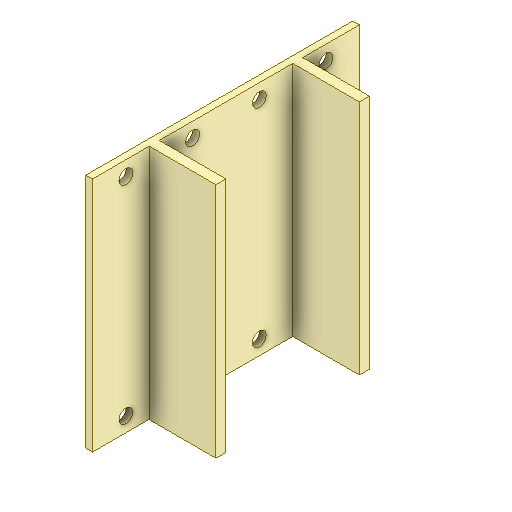
# Autodesk Inventor part: LegHolder
Saved by Autodesk Inventor 2022 (Build 260153000, 153)
## iProperties
Created: 2024-07-11
Part Number: LegHolder
Material: ABS Plastic
Document SubType Name: Modeling
Designer: LaptopJR
Density: 1.06 g/cm^3
Appearance: Nylon 6
Author: LaptopJR
Autodesk Inventor part; units mm, degrees
ref_plane "YZ Plane" through (0, 0, 0) normal (1, 0, 0) x (0, 1, 0)
ref_plane "XZ Plane" through (0, 0, 0) normal (0, 1, 0) x (-1, 0, 0)
ref_plane "Work Plane1" through (-4544.258, -3059.401, -4421.2024) normal (1, 0, 0) x (0, 1, 0)
sketch "Sketch1" plane through (-4544.258, -3059.401, -4421.2024) normal (1, 0, 0) x (0, 1, 0)
  line L0 (0.76, -160) -> (142.55, -160) projected
  line L1 (142.55, -160) -> (142.55, 0) projected
  line L2 (0.76, 0) -> (142.55, 0) projected
  line L3 (0.76, 0) -> (0.76, -160) projected
  arc A0 (9.505, -144.1656) -> (9.505, -135.8344) centre (9.505, -140) ccw projected
  arc A1 (9.505, -135.8344) -> (9.505, -144.1656) centre (9.505, -140) ccw projected
  arc A2 (133.805, -144.1656) -> (133.805, -135.8344) centre (133.805, -140) ccw projected
  arc A3 (133.805, -135.8344) -> (133.805, -144.1656) centre (133.805, -140) ccw projected
  arc A4 (133.805, -24.1656) -> (133.805, -15.8344) centre (133.805, -20) ccw projected
  arc A5 (133.805, -15.8344) -> (133.805, -24.1656) centre (133.805, -20) ccw projected
  arc A6 (9.505, -24.1656) -> (9.505, -15.8344) centre (9.505, -20) ccw projected
  arc A7 (9.505, -15.8344) -> (9.505, -24.1656) centre (9.505, -20) ccw projected
  arc A8 (51.655, -144.9403) -> (51.655, -135.0597) centre (51.655, -140) ccw construction
  arc A9 (51.655, -135.0597) -> (51.655, -144.9403) centre (51.655, -140) ccw construction
  arc A10 (51.655, -24.9403) -> (51.655, -15.0597) centre (51.655, -20) ccw construction
  arc A11 (51.655, -15.0597) -> (51.655, -24.9403) centre (51.655, -20) ccw construction
  arc A12 (91.655, -24.9403) -> (91.655, -15.0597) centre (91.655, -20) ccw construction
  arc A13 (91.655, -15.0597) -> (91.655, -24.9403) centre (91.655, -20) ccw construction
  arc A14 (9.505, -64.1656) -> (9.505, -55.8344) centre (9.505, -60) ccw projected
  arc A15 (9.505, -55.8344) -> (9.505, -64.1656) centre (9.505, -60) ccw projected
  arc A16 (9.505, -104.1656) -> (9.505, -95.8344) centre (9.505, -100) ccw projected
  arc A17 (9.505, -95.8344) -> (9.505, -104.1656) centre (9.505, -100) ccw projected
  arc A18 (133.805, -104.1656) -> (133.805, -95.8344) centre (133.805, -100) ccw projected
  arc A19 (133.805, -95.8344) -> (133.805, -104.1656) centre (133.805, -100) ccw projected
  arc A20 (133.805, -64.1656) -> (133.805, -55.8344) centre (133.805, -60) ccw projected
  arc A21 (133.805, -55.8344) -> (133.805, -64.1656) centre (133.805, -60) ccw projected
  arc A22 (51.655, -64.9403) -> (51.655, -55.0597) centre (51.655, -60) ccw construction
  arc A23 (51.655, -55.0597) -> (51.655, -64.9403) centre (51.655, -60) ccw construction
  arc A24 (51.655, -104.9403) -> (51.655, -95.0597) centre (51.655, -100) ccw construction
  arc A25 (51.655, -95.0597) -> (51.655, -104.9403) centre (51.655, -100) ccw construction
  arc A26 (91.655, -104.9403) -> (91.655, -95.0597) centre (91.655, -100) ccw construction
  arc A27 (91.655, -95.0597) -> (91.655, -104.9403) centre (91.655, -100) ccw construction
  arc A28 (91.655, -64.9403) -> (91.655, -55.0597) centre (91.655, -60) ccw construction
  arc A29 (91.655, -55.0597) -> (91.655, -64.9403) centre (91.655, -60) ccw construction
  arc A30 (91.655, -144.9403) -> (91.655, -135.0597) centre (91.655, -140) ccw construction
  arc A31 (91.655, -135.0597) -> (91.655, -144.9403) centre (91.655, -140) ccw construction
  point P0 (3059.401, 4421.2024)
extrude "Extrusion1" add sketch "Sketch1" along normal blind 4
sketch "Sketch2" plane through (-4540.258, -3059.401, -4421.2024) normal (1, 0, 0) x (0, 0, -1)
  line L0 (160, 142.55) -> (0, 142.55) projected
  line L1 (34, 0.5504) -> (40, 0.5504)
  line L2 (40, 0.5504) -> (40, 142.55)
  line L3 (40, 142.55) -> (34, 142.55)
  line L4 (34, 142.55) -> (34, 0.5504)
  line L5 (0, 0.76) -> (160, 0.76) projected
  line L6 (120, 0.76) -> (126, 0.76)
  line L7 (126, 0.76) -> (126, 142.55)
  line L8 (126, 142.55) -> (120, 142.55)
  line L9 (120, 142.55) -> (120, 0.76)
  line L10 (0, 142.55) -> (0, 0.76) projected
  point P0 (-4421.2024, 3059.401)
  point P1 (120, 142.55)
  point P2 (126, 0.76)
  point P3 (34, 142.55)
  dimension "d2" = 6
  dimension "d3" = 6
  dimension "d4" = 80
  dimension "d5" = 34
  constraints: 16 end point, 4 parallel, 3 point on line, 2 horizontal, 2 perpendicular
  measures "d2" distance between parallel lines of L2 L4
  measures "d3" distance between parallel lines of L7 L9
  measures "d4" distance between parallel lines of L9 L2
  measures "d5" distance between parallel lines of L10 L4
extrude "Extrusion2" add sketch "Sketch2" along normal blind 40 contours L7 L5 L9 L0 | L2 L5 L4 L0 | L2 L1 L4 L5
body "Solid1"
